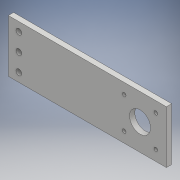
# Autodesk Inventor part: MotorPlateOld
Saved by Autodesk Inventor 2017 (Build 210142000, 142)
## iProperties
Created: 2017-03-12
Part Number: MotorPlateOld
Material: Generic
Document SubType Name: Modeling
Designer: umr
Density: 1 g/cm^3
Appearance: Default
Author: umr
Autodesk Inventor part; units mm, degrees
ref_plane "YZ Plane" through (0, 0, 0) normal (1, 0, 0) x (0, 1, 0)
ref_plane "XZ Plane" through (0, 0, 0) normal (0, 1, 0) x (-1, 0, 0)
ref_plane "XY Plane" through (0, 0, 0) normal (0, 0, 1) x (1, 0, 0)
sketch "Sketch1" plane through (0, 0, 0) normal (0, 1, 0) x (-1, 0, 0)
  line L0 (0, 0) -> (150, 0)
  line L1 (150, 0) -> (150, -50)
  line L2 (150, -50) -> (0, -50)
  line L3 (0, -50) -> (0, 0)
  dimension "d0" = 150
  dimension "d1" = 50
  constraints: 8 end point, 2 parallel, 1 horizontal, 1 perpendicular
  measures "d0" distance of L1.end L2.end
  measures "d1" distance of L0.end L1.end
extrude "Extrusion1" add sketch "Sketch1" along normal blind 5
sketch "Sketch2" plane through (0, 5, 0) normal (0, 1, 0) x (1, 0, 0)
  line L0 (-150, 0) -> (0, 0) projected
  line L1 (0, 0) -> (0, 50) projected
  line L2 (0, 50) -> (-150, 50) projected
  line L3 (-150, 50) -> (-150, 0) projected
  circle A0 centre (-140, 41.6667) radius 2.75
  circle A1 centre (-140, 25) radius 2.75
  circle A2 centre (-140, 8.3333) radius 2.75
  circle A3 centre (-40, 10) radius 1.75
  circle A4 centre (-40, 40) radius 1.75
  circle A5 centre (-10, 10) radius 1.75
  circle A6 centre (-10, 40) radius 1.75
  circle A7 centre (-25, 25) radius 10
  dimension "d4" = 5.5
  dimension "d5" = 50
  dimension "d6" = 8.3333
  dimension "d7" = 10
  dimension "d10" = 16.6667
  dimension "d16" = 3.5
  dimension "d19" = 30
  dimension "d22" = 30
  dimension "d25" = 10
  dimension "d26" = 10
  dimension "d27" = 20
  dimension "d28" = 25
  dimension "d29" = 25
  constraints: 8 centre point, 2 vertical, 1 horizontal, 10 other
  measures "d4" diameter of A0
  measures "d5" distance of L2.end L0.start
  measures "d6" distance from line of L2 A0.centre
  measures "d7" distance from line of L3 A0.centre
  measures "d10" distance of A0.centre A1.centre
  measures "d16" diameter of A3
  measures "d19" distance of A3.centre A4.centre
  measures "d22" distance of A3.centre A5.centre
  measures "d25" distance from line of L0 A3.centre
  measures "d26" distance from line of L1 A5.centre
  measures "d27" diameter of A7
  measures "d28" distance from line of L0 A7.centre
  measures "d29" distance from line of L1 A7.centre
extrude "Extrusion2" cut sketch "Sketch2" against normal blind 5 contours A0 | A1 | A2 | A3 | A4 | A5 | A6 | A7
equation "\"d6\" = 0.166667 * d5"
equation "\"d10\" = 2 * d6"
equation "\"d22\" = d19"
equation "\"d25\" = -0.5 * d19 + 0.5 * d5"
equation "\"d26\" = d25"
equation "\"d28\" = 0.5 * d5"
equation "\"d29\" = d28"
body "Solid1"
